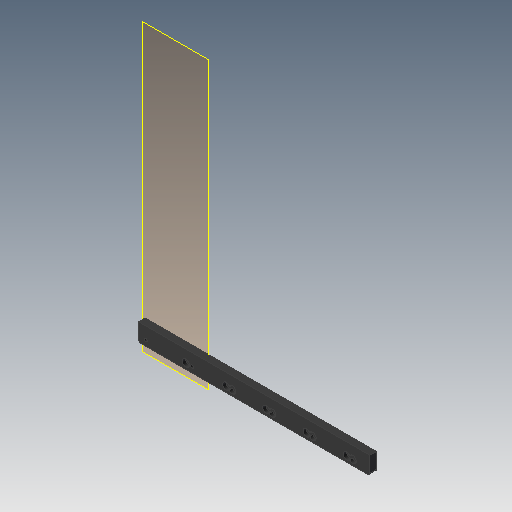
# Autodesk Inventor part: 03_Opentrons_Microscope_MTP_stand
Saved by Autodesk Inventor 2019.4 (Build 234330000, 330)
## iProperties
Created: 2020-10-28
Part Number: 03_Opentrons_Microscope_MTP_stand
Material: Generic
Document SubType Name: Modeling
Designer: diederichbenedict
Density: 1 g/cm^3
Appearance: Default
Author: diederichbenedict
Autodesk Inventor part; units mm, degrees
ref_plane "YZ Plane" through (0, 0, 0) normal (1, 0, 0) x (0, 1, 0)
ref_plane "XZ Plane" through (0, 0, 0) normal (0, 1, 0) x (-1, 0, 0)
ref_plane "XY Plane" through (0, 0, 0) normal (0, 0, 1) x (1, 0, 0)
ref_plane "Work Plane1" through (0, 0, 0) normal (0, 0, 1) x (1, 0, 0)
sketch "Sketch1" plane through (0, 0, 0) normal (0, 0, 1) x (1, 0, 0)
  circle A0 centre (-21, 106) radius 1.45 projected
  circle A1 centre (-21, 69.5) radius 1.45 projected
  circle A2 centre (-21, 33) radius 1.45 projected
  circle A3 centre (-21, -3.5) radius 1.45 projected
  circle A4 centre (-21, -40) radius 1.45 projected
  circle A5 centre (-21, -113) radius 1.45 projected
  circle A6 centre (21, -113) radius 1.45 projected
  circle A7 centre (21, -40) radius 1.45 projected
  circle A8 centre (21, -3.5) radius 1.45 projected
  circle A9 centre (21, 33) radius 1.45 projected
  circle A10 centre (21, 69.5) radius 1.45 projected
  circle A11 centre (21, 106) radius 1.45 projected
  arc A12 (-6.5, 102) -> (-11.5, 97) centre (-6.5, 97) ccw projected
  line L0 (-6.5, 102) -> (6.5, 102) projected
  arc A13 (11.5, 97) -> (6.5, 102) centre (6.5, 97) ccw projected
  line L1 (11.5, 97) -> (11.5, -97) projected
  arc A14 (6.5, -102) -> (11.5, -97) centre (6.5, -97) ccw projected
  line L2 (6.5, -102) -> (-6.5, -102) projected
  arc A15 (-11.5, -97) -> (-6.5, -102) centre (-6.5, -97) ccw projected
  line L3 (-11.5, -97) -> (-11.5, 97) projected
  arc A16 (25.5, -118) -> (27.5, -116) centre (25.5, -116) ccw projected
  line L4 (27.5, -116) -> (27.5, 116) projected
  arc A17 (27.5, 116) -> (25.5, 118) centre (25.5, 116) ccw projected
  line L5 (25.5, 118) -> (-25.5, 118) projected
  arc A18 (-25.5, 118) -> (-27.5, 116) centre (-25.5, 116) ccw projected
  line L6 (-27.5, 116) -> (-27.5, -116) projected
  arc A19 (-27.5, -116) -> (-25.5, -118) centre (-25.5, -116) ccw projected
  line L7 (-25.5, -118) -> (25.5, -118) projected
  circle A20 centre (21, -76.5) radius 1.45 projected
  circle A21 centre (-21, -76.5) radius 1.45 projected
  circle A22 centre (21, 111.5) radius 1.45 projected
  circle A23 centre (-21, 111.5) radius 1.45 projected
  arc A24 (48.8107, 3.6492) -> (48.6958, 3.3718) centre (50.5958, 2.7473) ccw construction
  line L8 (48.6958, -66.1718) -> (48.6958, 3.3718) construction
  arc A25 (48.6958, -66.1718) -> (48.8107, -66.4492) centre (50.5958, -65.5473) ccw construction
  line L9 (54.3466, -71.9851) -> (48.8107, -66.4492) construction
  arc A26 (54.3466, -71.9851) -> (54.624, -72.1) centre (55.2485, -70.2) ccw construction
  line L10 (170.6958, -72.1) -> (54.624, -72.1) construction
  arc A27 (170.6958, -72.1) -> (172.2958, -70.5) centre (170.6958, -70.5) ccw construction
  line L11 (172.2958, 7.7) -> (172.2958, -70.5) construction
  arc A28 (172.2958, 7.7) -> (170.6958, 9.3) centre (170.6958, 7.7) ccw construction
  line L12 (54.624, 9.3) -> (170.6958, 9.3) construction
  arc A29 (54.624, 9.3) -> (54.3466, 9.1851) centre (55.2485, 7.4) ccw construction
  line L13 (48.8107, 3.6492) -> (54.3466, 9.1851) construction
  line L14 (56.1958, 4.9) -> (164.7958, 4.9) construction
  line L15 (164.7958, 4.9) -> (164.7958, -67.7) construction
  line L16 (164.7958, -67.7) -> (56.1958, -67.7) construction
  line L17 (56.1958, -67.7) -> (56.1958, 4.9) construction
  line L18 (174.3958, -70.2) -> (174.3958, 7.4) construction
  arc A30 (50.5958, 11.1) -> (46.8958, 7.4) centre (50.5958, 7.4) ccw construction
  arc A31 (46.6958, -70.2) -> (50.5958, -74.1) centre (50.5958, -70.2) ccw construction
  arc A32 (174.2958, 7.4) -> (170.3958, 11.3) centre (170.3958, 7.4) ccw construction
  arc A33 (170.3958, -74.1) -> (174.2958, -70.2) centre (170.3958, -70.2) ccw construction
  line L19 (-27.5, -118) -> (182.5, -118)
  line L20 (182.5, -118) -> (182.5, -102)
  line L21 (182.5, -102) -> (-27.5, -102)
  line L22 (-27.5, -102) -> (-27.5, -118)
  circle A34 centre (21, -113) radius 1.45 construction
  circle A35 centre (-21, -113) radius 1.45 construction
  line L23 (27.5, -102) -> (11.5, -102)
  line L24 (11.5, -102) -> (11.5, -70)
  line L25 (11.5, -70) -> (27.5, -70)
  line L26 (27.5, -70) -> (27.5, -102)
  line L27 (-27.5, -102) -> (-11.5, -102)
  line L28 (-11.5, -102) -> (-11.5, -70)
  line L29 (-11.5, -70) -> (-27.5, -70)
  line L30 (-27.5, -70) -> (-27.5, -102)
  circle A36 centre (21, -76.5) radius 1.45 projected
  circle A37 centre (-21, -76.5) radius 1.45 projected
  circle A38 centre (21, -113) radius 1.45 projected
  circle A39 centre (-21, -113) radius 1.45 projected
  circle A40 centre (21, -113) radius 1.45
  circle A41 centre (-21, -113) radius 1.45
  circle A42 centre (15.5, -113) radius 1.45
  circle A43 centre (57.5, -113) radius 1.45
  circle A44 centre (52, -113) radius 1.45
  circle A45 centre (94, -113) radius 1.45
  circle A46 centre (88.5, -113) radius 1.45
  circle A47 centre (130.5, -113) radius 1.45
  circle A48 centre (125, -113) radius 1.45
  circle A49 centre (167, -113) radius 1.45
  circle A50 centre (161.5, -113) radius 1.45
  circle A51 centre (203.5, -113) radius 1.45
  circle A52 centre (198, -113) radius 1.45
  circle A53 centre (240, -113) radius 1.45
  circle A54 centre (234.5, -113) radius 1.45
  circle A55 centre (276.5, -113) radius 1.45
  circle A56 centre (271, -113) radius 1.45
  circle A57 centre (313, -113) radius 1.45
  circle A58 centre (307.5, -113) radius 1.45
  circle A59 centre (349.5, -113) radius 1.45
  point P0 (0, 0)
  dimension "d1" = 210
  dimension "d2" = 32
  dimension "d8" = 36.5
  constraints: 24 end point, 20 centre point, 20 coincident, 6 parallel, 5 point on line, 4 horizontal, 3 perpendicular, 2 concentric, 90 other
  measures "d1" distance of L21.end L20.end
  measures "d2" distance of L23.end L24.end
  measures "d8" distance of A6.centre point (57.5, -113)
extrude "Extrusion1" add sketch "Sketch1" along normal blind 6 contours L2 L21 L4 A16 L7 A19 L6 | A19 L19 L22 | L21 L20 L19 A16 L4 | A42 | A43 | A44 | A45 | A46 | A47 | A48 | A49 | A50
fillet "Fillet1" radius 2 2 edges at (-27.5, -118, 3) (182.5, -118, 3)
sketch "Sketch2" plane through (0, 0, 6) normal (0, 0, 1) x (1, 0, 0)
  arc A0 (180.5, -118) -> (182.5, -116) centre (180.5, -116) ccw projected
  line L0 (182.5, -116) -> (182.5, -102) projected
  line L1 (182.5, -102) -> (-27.5, -102) projected
  line L2 (-27.5, -102) -> (-27.5, -116) projected
  arc A1 (-27.5, -116) -> (-25.5, -118) centre (-25.5, -116) ccw projected
  line L3 (-25.5, -118) -> (180.5, -118) projected
  line L4 (-25.1, -118) -> (-25.1, -108)
  point P0 (0, 0)
  point P1 (57.5, -113)
  point P2 (15.5, -113)
  point P3 (94, -113)
  point P4 (52, -113)
  point P5 (130.5, -113)
  point P6 (88.5, -113)
  point P7 (167, -113)
  point P8 (125, -113)
  point P9 (203.5, -113)
  point P10 (161.5, -113)
  point P11 (240, -113)
  point P12 (198, -113)
  point P13 (276.5, -113)
  point P14 (234.5, -113)
  point P15 (313, -113)
  point P16 (271, -113)
  point P17 (349.5, -113)
  point P18 (307.5, -113)
  dimension "d15" = 36.5
  constraints: 2 end point, 1 horizontal, 1 vertical, 18 other
hole "Hole1" at (15.5, -113, 6) at (52, -113, 6) at (57.5, -113, 6) at (88.5, -113, 6) at (94, -113, 6) at (125, -113, 6) at (130.5, -113, 6) at (161.5, -113, 6) at (167, -113, 6) direction (0, 0, -1) diameter 2.9 end through all counterbore diameter 6.5 counterbore depth 3
body "Solid1"
